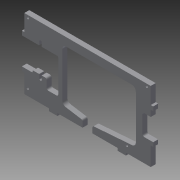
# Autodesk Inventor part: MainPanel5
Saved by Autodesk Inventor 2015 (Build 190159000, 159)
## iProperties
Created: 2014-08-06
Part Number: MainPanel5
Material: Generic
Document SubType Name: Modeling
Designer: STACKPOLE
Density: 1 g/cm^3
Appearance: Default
Author: STACKPOLE
Autodesk Inventor part; units mm, degrees
ref_plane "YZ Plane" through (0, 0, 0) normal (1, 0, 0) x (0, 1, 0)
ref_plane "XZ Plane" through (0, 0, 0) normal (0, 1, 0) x (-1, 0, 0)
ref_plane "XY Plane" through (0, 0, 0) normal (0, 0, 1) x (1, 0, 0)
sketch "Sketch1" plane through (0, 0, 0) normal (0, 1, 0) x (-1, 0, 0)
  line L0 (153, 85) -> (0, 85)
  line L1 (0, 65) -> (-3, 65)
  line L2 (-3, 65) -> (-3, 60)
  line L3 (-3, 60) -> (0, 60)
  line L4 (0, 40) -> (153, 40) construction
  line L5 (0, 27.5) -> (-3, 27.5)
  line L6 (-3, 27.5) -> (-3, 22.5)
  line L7 (-3, 22.5) -> (0, 22.5)
  line L8 (153, 65) -> (156, 65)
  line L9 (156, 65) -> (156, 60)
  line L10 (156, 60) -> (153, 60)
  line L11 (153, 27.5) -> (156, 27.5)
  line L12 (156, 27.5) -> (156, 22.5)
  line L13 (156, 22.5) -> (153, 22.5)
  line L14 (153, 65) -> (153, 85)
  line L15 (153, 0) -> (153, 22.5)
  line L16 (153, 27.5) -> (153, 60)
  line L17 (0, 85) -> (0, 65)
  line L18 (0, 60) -> (0, 27.5)
  line L19 (0, 22.5) -> (0, 0)
  line L20 (40, 0) -> (40, -3)
  line L21 (40, -3) -> (30, -3)
  line L22 (30, -3) -> (30, 0)
  line L23 (123, 0) -> (123, -3)
  line L24 (123, -3) -> (113, -3)
  line L25 (113, -3) -> (113, 0)
  line L26 (0, 0) -> (30, 0)
  line L27 (40, 0) -> (113, 0)
  line L28 (123, 0) -> (153, 0)
  dimension "d0" = 85
  dimension "d1" = 153
  dimension "d3" = 3
  dimension "d4" = 20
  dimension "d5" = 5
  dimension "d6" = 3
  dimension "d7" = 12.5
  dimension "d9" = 3
  dimension "d10" = 5
  dimension "d11" = 3
  dimension "d12" = 12.5
  dimension "d13" = 20
  dimension "d16" = 20
  dimension "d39" = 10
  dimension "d40" = 3
  dimension "d41" = 10
  dimension "d42" = 3
  dimension "d43" = 30
  dimension "d44" = 30
  dimension "d66" = 5
  dimension "d67" = 5
  constraints: 58 end point, 18 parallel, 13 perpendicular, 9 horizontal, 4 vertical alignment, 2 horizontal alignment, 2 point on line
  measures "d0" distance of L0.end L19.end
  measures "d1" distance of L19.end L15.start
  measures "d3" distance of L1.start L1.end
  measures "d4" distance between parallel lines of L4 L3
  measures "d5" distance of L5.end L6.end
  measures "d6" distance of L6.end L7.end
  measures "d7" distance between parallel lines of L4 L5
  measures "d9" distance of L8.start L8.end
  measures "d10" distance of L11.end L12.end
  measures "d11" distance of L12.end L13.end
  measures "d12" distance between parallel lines of L4 L11
  measures "d13" distance between parallel lines of L4 L10
  measures "d16" distance between parallel lines of L0 L1
  measures "d39" distance of L20.end L21.end
  measures "d40" distance of L20.start L20.end
  measures "d41" distance of L23.end L24.end
  measures "d42" distance of L24.end L25.end
  measures "d43" distance between parallel lines of L15 L23
  measures "d44" distance between parallel lines of L19 L22
  measures "d66" distance of L1.end L2.end
  measures "d67" distance of L8.end L9.end
extrude "Extrusion1" add sketch "Sketch1" along normal blind 6
sketch "Sketch2" plane through (0, 6, 0) normal (0, 1, 0) x (1, 0, 0)
  line L0 (-153, -27.5) -> (-153, -60) projected
  line L1 (0, -60) -> (0, -27.5) projected
  line L2 (-143, -30) -> (-135, -30)
  line L3 (-135, -60) -> (-153, -60)
  line L4 (-135, -24) -> (-132, -24)
  line L5 (-132, -66) -> (-135, -66)
  line L6 (-132, -30) -> (-128, -30)
  line L7 (-112, -60) -> (-132, -60)
  line L8 (-132, -24) -> (-132, -30)
  line L9 (-132, -60) -> (-132, -66)
  line L10 (-135, -66) -> (-135, -60)
  line L11 (-135, -30) -> (-135, -24)
  line L12 (-153, -60) -> (-153, -30)
  line L13 (-126, -28) -> (-126, -20)
  line L14 (-124, -18) -> (-114, -18)
  arc A0 (-128, -30) -> (-126, -28) centre (-128, -28) ccw
  arc A1 (-124, -18) -> (-126, -20) centre (-124, -20) ccw
  arc A2 (-112, -20) -> (-114, -18) centre (-114, -20) ccw
  line L15 (-112, -60) -> (-112, -20)
  line L16 (-156, -27.5) -> (-153, -27.5) projected
  line L17 (-153, -40) -> (0, -40) construction
  line L18 (3, -22.5) -> (0, -22.5) projected
  line L19 (-153, -27.5) -> (-143, -27.5)
  line L20 (-143, -27.5) -> (-143, -30)
  dimension "d22" = 42
  dimension "d24" = 3
  dimension "d26" = 6
  dimension "d47" = 2
  dimension "d69" = 20
  dimension "d71" = 12.5
  dimension "d72" = 10
  dimension "d73" = 20
  dimension "d74" = 6
  dimension "d96" = 42
  dimension "d97" = 10
  dimension "d122" = 41
  dimension "d123" = 6
  constraints: 34 end point, 8 parallel, 6 point on circle, 6 tangent, 4 perpendicular, 3 centre point, 3 horizontal, 3 point on line, 2 equal radius, 2 vertical alignment, 1 collinear, 1 horizontal alignment
  measures "d22" distance between parallel lines of L5 L4
  measures "d24" distance of L4.start L4.end
  measures "d26" distance between parallel lines of L7 L5
  measures "d47" radius of A0
  measures "d69" distance between parallel lines of L15 L9
  measures "d71" distance between parallel lines of L17 L16
  measures "d72" distance between parallel lines of L17 L2
  measures "d73" distance between parallel lines of L3 L17
  measures "d74" distance of L2.end L4.start
  measures "d96" distance between parallel lines of L7 L14
  measures "d97" distance of L0.start L19.end
  measures "d122" distance between parallel lines of L0 L15
  measures "d123" distance between parallel lines of L8 L13
extrude "Extrusion2" cut sketch "Sketch2" against normal through all
sketch "Sketch3" plane through (0, 6, 0) normal (0, 1, 0) x (1, 0, 0)
  line L0 (-153, -85) -> (0, -85)
  line L1 (0, -60) -> (0, -27.5)
  line L2 (0, 0) -> (-153, 0)
  line L3 (-18, -16.633539) -> (-18, -70)
  line L4 (-23, -75) -> (-102, -75)
  line L5 (-107, -70) -> (-107, -16.249874)
  arc A0 (-23, -75) -> (-18, -70) centre (-23, -70) ccw
  arc A1 (-107, -70) -> (-102, -75) centre (-102, -70) ccw
  line L6 (0, -22.5) -> (0, 0)
  arc A2 (-18, -12) -> (-18, -12) centre (-18, -12) ccw
  arc A3 (-107, -12) -> (-107, -12) centre (-107, -12) ccw
  line L7 (-82.5, -8) -> (-82.5, 0)
  line L8 (-82.5, 0) -> (-70.5, 0)
  line L9 (-70.5, 0) -> (-70.5, -8)
  line L10 (-113, 0) -> (-113, 3)
  line L11 (-22.620149, -11.647989) -> (-70.5, -8)
  line L12 (-82.5, -8) -> (-102.805659, -11.31521)
  arc A4 (-18, -16.633539) -> (-22.620149, -11.647989) centre (-23, -16.633539) ccw
  arc A5 (-102.805659, -11.31521) -> (-107, -16.249874) centre (-102, -16.249874) ccw
  point P0 (0, -6)
  point P1 (-123, 0)
  dimension "d34" = 10
  dimension "d35" = 18
  dimension "d107" = 89
  dimension "d114" = 12
  dimension "d115" = 30.5
  dimension "d116" = 12
  dimension "d127" = 8
  dimension "d128" = 8
  constraints: 16 end point, 10 tangent, 8 point on circle, 7 point on line, 6 centre point, 4 coincident with centre, 2 parallel, 1 horizontal alignment
  measures "d34" distance between parallel lines of L0 L4
  measures "d35" distance between parallel lines of L1 L3
  measures "d107" distance between parallel lines of L3 L5
  measures "d114" distance between parallel lines of L9 L7
  measures "d115" distance between parallel lines of L10 L7
  measures "d116" distance from line of L2 A2.centre
  measures "d127" distance of L8.end L9.end
  measures "d128" distance of L7.start L7.end
sketch "Sketch6" plane through (0, 0, 0) normal (0, -1, 0) x (1, 0, 0)
  line L0 (0, 27.5) -> (0, 60)
  line L1 (-156, 60) -> (-135, 60)
  line L2 (0, 52.5) -> (-10, 52.5)
  line L3 (-10, 52.5) -> (-10, 27.5)
  line L4 (-10, 27.5) -> (0, 27.5)
  line L5 (0, 27.5) -> (0, 52.5)
  line L6 (0, 40) -> (-253.911448, 40) construction
  point P0 (-140, 60)
  dimension "d75" = 25
  dimension "d77" = 20
  dimension "d78" = 10
  constraints: 10 end point, 2 parallel, 2 perpendicular, 1 horizontal, 1 midpoint, 1 point on line
  measures "d75" distance of L4.end L2.start
  measures "d77" distance between parallel lines of L6 L1
  measures "d78" distance of L2.start L2.end
extrude "Extrusion5" cut sketch "Sketch6" against normal blind 10
fillet "Fillet2" radius 2 2 edges at (-10, 3, 52.5) (-10, 3, 27.5)
fillet "Fillet3" radius 1 5 edges at (-112, 3, 60) (-132, 3, 66) (-135, 3, 66) (-135, 3, 24) (-132, 3, 24)
sketch "Sketch7" plane through (0, 0, 0) normal (0, -1, 0) x (1, 0, 0)
  line L0 (0, 85) -> (-153, 85) projected
  line L1 (-153, 85) -> (-153, 65) projected
  circle A0 centre (-149, 82) radius 1.5
  circle A1 centre (-149, 8) radius 1.5
  circle A2 centre (-5, 82) radius 1.5
  circle A3 centre (-29, 8) radius 1.5
  dimension "d84" = 3
  dimension "d86" = 4
  dimension "d87" = 3
  dimension "d88" = 3
  dimension "d89" = 74
  dimension "d90" = 3
  dimension "d91" = 144
  dimension "d92" = 3
  dimension "d93" = 24
  constraints: 4 centre point, 2 horizontal alignment, 1 vertical alignment
  measures "d84" diameter of A0
  measures "d86" distance from line of L1 A0.centre
  measures "d87" distance from line of L0 A0.centre
  measures "d88" diameter of A1
  measures "d89" distance between centres of A0 A1
  measures "d90" diameter of A2
  measures "d91" distance of A0.centre A2.centre
  measures "d92" diameter of A3
  measures "d93" horizontal distance of A3.centre A2.centre
extrude "Extrusion6" cut sketch "Sketch7" against normal through all
sketch "Sketch3 outline for Extrusion8" plane through (0, 6, 0) normal (0, 1, 0) x (1, 0, 0)
  line L0 (-102, -75) -> (-23, -75)
  arc A0 (-107, -70) -> (-102, -75) centre (-102, -70) ccw
  line L1 (-107, -16.249874) -> (-107, -70)
  arc A1 (-102.805659, -11.31521) -> (-107, -16.249874) centre (-102, -16.249874) ccw
  line L2 (-82.5, -8) -> (-102.805659, -11.31521)
  line L3 (-82.5, 0) -> (-82.5, -8)
  line L4 (-70.5, 0) -> (-82.5, 0)
  line L5 (-70.5, -8) -> (-70.5, 0)
  line L6 (-22.620149, -11.647989) -> (-70.5, -8)
  arc A2 (-18, -16.633539) -> (-22.620149, -11.647989) centre (-23, -16.633539) ccw
  line L7 (-18, -70) -> (-18, -16.633539)
  arc A3 (-23, -75) -> (-18, -70) centre (-23, -70) ccw
extrude "Extrusion8" cut sketch "Sketch3 outline for Extrusion8" against normal through all
fillet "Fillet8" radius 1 2 edges at (-143, 3, 30) (-143, 3, 27.5)
fillet "Fillet9" radius 0.5 2 edges at (-135, 3, 60) (-135, 3, 30)
fillet "Fillet10" radius 2 2 edges at (-82.5, 3, 8) (-70.5, 3, 8)
body "Solid1"
